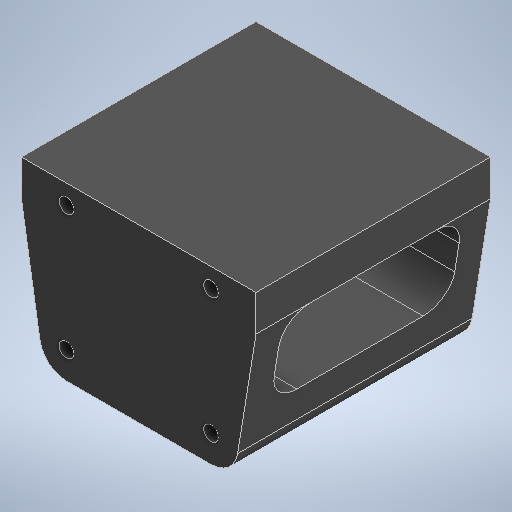
# Autodesk Inventor part: arm_middle
Saved by Autodesk Inventor 2026.1 (Build 301233020, 233B)
## iProperties
Created: 2024-02-14
Part Number: arm_middle
Material: 一般
Document SubType Name: Modeling
Designer: hibik
Density: 1 g/cm^3
Appearance: 既定
Author: hibik
Autodesk Inventor part; units mm, degrees
ref_plane "YZ Plane" through (0, 0, 0) normal (1, 0, 0) x (0, 1, 0)
ref_plane "XZ Plane" through (0, 0, 0) normal (0, 1, 0) x (-1, 0, 0)
ref_plane "XY Plane" through (0, 0, 0) normal (0, 0, 1) x (1, 0, 0)
sketch "スケッチ3" plane through (0, 0, 0) normal (1, 0, 0) x (0, 1, 0)
  line L0 (0, 0) -> (4, 0)
  line L1 (4, 0) -> (4, -26)
  line L2 (4, -26) -> (0, -26)
  line L3 (0, -26) -> (0, 0)
  line L4 (4, 0) -> (0, 0)
  line L5 (0, 0) -> (0, -26)
  line L6 (0, -26) -> (4, -26)
  line L7 (4, -26) -> (4, 0)
  line L8 (0, 0) -> (-15, 0)
  line L9 (-15, 0) -> (-15, -26)
  line L10 (-15, -26) -> (0, -26)
  line L11 (0, -26) -> (0, 0)
  dimension "d3" = 26
  dimension "d4" = 4
  dimension "d49" = 15
  constraints: 24 end point, 6 parallel, 3 horizontal, 3 perpendicular, 2 collinear, 1 point on line
  measures "d3" distance of L0.end L1.end
  measures "d4" distance between parallel lines of L1 L5
  measures "d49" distance of L4.end L8.end
extrude "押し出し2" add sketch "スケッチ3" along normal blind 26
sketch "スケッチ11" plane through (0, -15, 0) normal (0, 0, 1) x (1, 0, 0)
  circle A0 centre (5, 16.8437) radius 0.8 projected
  circle A1 centre (21, 16.8437) radius 0.8 projected
  point P0 (0, 15)
extrude "押し出し11" cut sketch "スケッチ11" against normal through all
sketch "スケッチ12" plane through (26, 0, 0) normal (1, 0, 0) x (0, 0, -1)
  line L0 (0, 4) -> (0, -15) projected
  line L1 (3, 0) -> (3, -9)
  line L2 (3, -9) -> (23, -9)
  line L3 (23, -9) -> (23, 0)
  line L4 (3, 0) -> (23, 0)
  line L5 (26, 4) -> (0, 4) projected
  line L6 (0, -15) -> (26, -15) projected
  point P0 (0, 0)
  point P1 (0, -0.1563)
  point P2 (13, 4)
  point P3 (13, 0)
  dimension "d62" = 3
  dimension "d63" = 6
  constraints: 8 end point, 2 horizontal, 2 midpoint, 2 point on line, 2 vertical, 1 vertical alignment
  measures "d62" distance from line of L0 L1.start
  measures "d63" distance between parallel lines of L6 L2
extrude "押し出し12" cut sketch "スケッチ12" against normal through all
fillet "フィレット1" radius 3 4 edges at (13, 0, -23) (13, 0, -3) (13, -9, -23) (13, -9, -3)
sketch "スケッチ13" plane through (0, -15, 0) normal (0, 0, 1) x (1, 0, 0)
  line L0 (0, 15) -> (2.4503, 0)
  line L1 (0, 0) -> (26, 0) projected
  line L2 (26, 12) -> (26, 15) projected
  line L3 (26, 15) -> (23.5494, -0.0019)
  circle A0 centre (5, 3) radius 3
  circle A1 centre (21, 3) radius 3
  line L4 (0, 0) -> (26, 0) projected
  line L5 (0, 19) -> (26, 19) projected
  line L6 (13, 19) -> (13, 0)
  circle A2 centre (5, 3) radius 0.8
  circle A3 centre (21, 3) radius 0.8
  circle A4 centre (5, 16.8437) radius 0.8 projected
  circle A5 centre (21, 16.8437) radius 0.8 projected
  line L7 (0, 19) -> (0, 0) projected
  line L8 (0, 0) -> (26, 0) projected
  line L9 (26, 19) -> (26, 0) projected
  line L10 (0, 19) -> (26, 19) projected
  point P0 (5, 0)
  point P1 (2.0392, 2.5164)
  point P2 (23.9608, 2.5164)
  point P3 (21, 0)
  dimension "d64" = 16
  dimension "d65" = 6
  dimension "d66" = 1.6
  dimension "d67" = 1.6
  constraints: 6 end point, 4 centre point, 2 coincident, 2 tangent, 1 equal radius, 1 midpoint, 1 point on line, 5 other
  measures "d64" distance of A1.centre A0.centre
  measures "d65" diameter of A0
  measures "d66" diameter of A2
  measures "d67" diameter of A3
extrude "押し出し13" cut sketch "スケッチ13" against normal through all contours L0 L1 L7 | A0 L1 L0 | A1 L3 L1 | L2 L9 L1 L3 | A2 | A3
